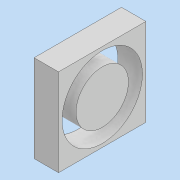
# Autodesk Inventor part: P00173-09-008
Saved by Autodesk Inventor 2022 (Build 260153070, 153G)
## iProperties
Created: 2021-04-13
Part Number: P00173-09-008
Material: Generic
Document SubType Name: Modeling
Designer: MPM
Density: 1 g/cm^3
Appearance: Default
Description: SUNON AXIAL FAN 5V
Stock Number: MF25060V2
Author: MPM
Comments: M2-Paypad 3d files for a Cardano blockchain payment terminal. Copyright (C) 2021 Maarten Menheere This program is free software; you can redistribute it and/or modify it under the terms of the GNU General Public License as published by the Free Software Foundation; either version 2 of the License, or (at your option) any later version. This program is distributed in the hope that it will be useful, but WITHOUT ANY WARRANTY; without even the implied warranty of MERCHANTABILITY or FITNESS FOR A PARTICULAR PURPOSE.  See the GNU General Public License for more details. You should have received a copy of the GNU General Public License along with this program; if not, write to the Free Software Foundation, Inc., 51 Franklin Street, Fifth Floor, Boston, MA  02110-1301, USA.
Autodesk Inventor part; units mm, degrees
ref_plane "YZ Plane" through (0, 0, 0) normal (1, 0, 0) x (0, 1, 0)
ref_plane "XZ Plane" through (0, 0, 0) normal (0, 1, 0) x (-1, 0, 0)
derived "P00173-09-002.ipt"
sketch "Fan_Side" plane through (-55.0091, 51.5, 7.4) normal (0, 1, 0) x (-1, 0, 0)
  line L0 (-1, 37) -> (-8, 37)
  line L1 (-8, 37) -> (-8, 12)
  line L2 (-8, 12) -> (-1, 12)
  line L3 (-1, 12) -> (-1, 37)
  point P0 (-55.0091, -7.4)
  point P1 (0, 0)
  point P2 (0, 0)
  point P3 (0, 0)
ref_plane "Work Plane2" through (-47.0091, 51.5, 19.4) normal (-1, 0, 0) x (0, -1, 0)
sketch "Sketch3" plane through (-47.0091, 51.5, 19.4) normal (-1, 0, 0) x (0, -1, 0)
  line L0 (0, 25) -> (0, 0) projected
  circle A0 centre (0, 12.5) radius 11.5
  circle A1 centre (0, 12.5) radius 7.5
  point P0 (51.5, -19.4)
  point P1 (0, 1)
  dimension "d7" = 1
  dimension "d8" = 4
  constraints: 1 centre point, 1 coincident, 1 midpoint, 1 point on line, 1 vertical alignment, 2 other
  measures "d7" distance of L0.end point (0, 1)
extrude "Extrusion2" add sketch "Fan_Side" along normal mid plane 25
extrude "Extrusion3" cut sketch "Sketch3" along normal blind 10 contours A0 L0 A1 | L0 A1 A0
ref_plane "Work Plane16" through (-55.0091, 51.5, 7.4) normal (0, 1, 0) x (-1, 0, 0)
body "Solid2"
